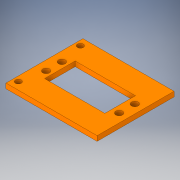
# Autodesk Inventor part: Pinza_sostenedor
Saved by Autodesk Inventor 2019 (Build 230136000, 136)
## iProperties
Created: 2020-02-07
Part Number: Pinza_sostenedor
Material: Generic
Document SubType Name: Modeling
Designer: Omar
Density: 1 g/cm^3
Appearance: Default
Author: Omar
Autodesk Inventor part; units mm, degrees
ref_plane "YZ Plane" through (0, 0, 0) normal (1, 0, 0) x (0, 1, 0)
ref_plane "XZ Plane" through (0, 0, 0) normal (0, 1, 0) x (-1, 0, 0)
ref_plane "XY Plane" through (0, 0, 0) normal (0, 0, 1) x (1, 0, 0)
sketch "Sketch1" plane through (0, 0, 0) normal (0, 1, 0) x (-1, 0, 0)
  line L0 (-19.5, 9.9) -> (19.5, 9.9)
  line L1 (19.5, 9.9) -> (19.5, -9.9)
  line L2 (19.5, -9.9) -> (-19.5, -9.9)
  line L3 (-19.5, -9.9) -> (-19.5, 9.9)
  line L4 (-19.5, 9.9) -> (19.5, -9.9) construction
  line L5 (19.5, 9.9) -> (-19.5, -9.9) construction
  line L6 (29.5, 24.9) -> (-29.5, 24.9)
  line L7 (-29.5, 24.9) -> (-29.5, -24.9)
  line L8 (-29.5, -24.9) -> (29.5, -24.9)
  line L9 (29.5, -24.9) -> (29.5, 24.9)
  circle A0 centre (23.31, -5.085) radius 2.19
  circle A1 centre (23.31, 5.085) radius 2.19
  circle A2 centre (-23.95, 5.085) radius 2.19
  circle A3 centre (-23.95, -5.085) radius 2.19
  circle A4 centre (26.31, 20.085) radius 1.905
  circle A5 centre (26.31, -20.085) radius 1.905
  point P0 (0, 0)
  dimension "d0" = 39
  dimension "d1" = 19.8
  dimension "d2" = 10
  dimension "d3" = 10
  dimension "d4" = 15
  dimension "d5" = 15
  dimension "d6" = 4.38
  dimension "d7" = 4.38
  dimension "d8" = 5.085
  dimension "d9" = 5.085
  dimension "d10" = 3.81
  dimension "d11" = 3.81
  dimension "d12" = 47.26
  dimension "d13" = 47.26
  dimension "d14" = 4.38
  dimension "d15" = 4.38
  dimension "d16" = 5.085
  dimension "d17" = 5.085
  dimension "d18" = 3.81
  dimension "d19" = 3.81
  dimension "d20" = 15
  dimension "d21" = 15
  dimension "d22" = 3
  dimension "d23" = 3
  constraints: 20 end point, 6 centre point, 4 parallel, 2 horizontal, 2 midpoint, 2 perpendicular
  measures "d0" distance of L1.end L2.end
  measures "d1" distance of L0.end L1.end
  measures "d2" distance between parallel lines of L9 L1
  measures "d3" distance between parallel lines of L3 L7
  measures "d4" distance between parallel lines of L2 L8
  measures "d5" distance between parallel lines of L6 L0
  measures "d6" diameter of A1
  measures "d7" diameter of A0
  measures "d8" vertical distance of A0.centre point (0, 0)
  measures "d9" vertical distance of point (0, 0) A1.centre
  measures "d10" distance from line of L1 A0.centre
  measures "d11" distance from line of L1 A1.centre
  measures "d12" distance of A1.centre A2.centre
  measures "d13" distance of A3.centre A0.centre
  measures "d14" diameter of A3
  measures "d15" diameter of A2
  measures "d16" vertical distance of A2.centre point (0, 0)
  measures "d17" vertical distance of point (0, 0) A3.centre
  measures "d18" diameter of A4
  measures "d19" diameter of A5
  measures "d20" vertical distance of A4.centre A1.centre
  measures "d21" vertical distance of A0.centre A5.centre
  measures "d22" horizontal distance of A5.centre A0.centre
  measures "d23" horizontal distance of A1.centre A4.centre
extrude "Extrusion1" add sketch "Sketch1" along normal blind 3.18
body "Solid1"
